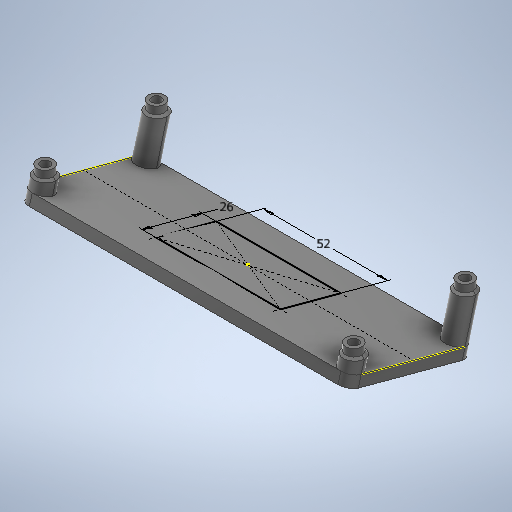
# Autodesk Inventor part: relay_module_standoffs_angled_plate
Saved by Autodesk Inventor 2025.1 (Build 291241000, 241)
## iProperties
Created: 2026-06-20
Part Number: relay_module_standoffs_angled_plate
Material: Generic
Document SubType Name: Modeling
Designer: Aiden
Density: 1 g/cm^3
Appearance: Default
Author: Aiden
Autodesk Inventor part; units mm, degrees
ref_plane "YZ Plane" through (0, 0, 0) normal (1, 0, 0) x (0, 1, 0)
ref_plane "XZ Plane" through (0, 0, 0) normal (0, 1, 0) x (-1, 0, 0)
ref_plane "XY Plane" through (0, 0, 0) normal (0, 0, 1) x (1, 0, 0)
sketch "Relay Hole Layout" plane through (0, 0, 0) normal (0, 1, 0) x (-1, 0, 0)
  line L0 (64.4668, 23.2607) -> (-64.4668, 23.2607) construction
  line L1 (-64.4668, 23.2607) -> (-64.4668, -23.2607) construction
  line L2 (-64.4668, -23.2607) -> (64.4668, -23.2607) construction
  line L3 (64.4668, -23.2607) -> (64.4668, 23.2607) construction
  line L4 (64.4668, 23.2607) -> (-64.4668, -23.2607) construction
  line L5 (-64.4668, 23.2607) -> (64.4668, -23.2607) construction
  circle A0 centre (64.4668, -23.2607) radius 1.625 construction
  line L6 (0, -23.2607) -> (0, 23.2607) construction
  line L7 (64.4668, 0) -> (-64.4668, 0) construction
  circle A1 centre (-64.4668, -23.2607) radius 1.625 construction
  circle A2 centre (64.4668, 23.2607) radius 1.625 construction
  circle A3 centre (-64.4668, 23.2607) radius 1.625 construction
  line L8 (67.4918, -26.2857) -> (-67.4918, -26.2857) construction
  line L9 (-67.4918, -26.2857) -> (-67.4918, 26.2857) construction
  line L10 (-67.4918, 26.2857) -> (67.4918, 26.2857) construction
  line L11 (67.4918, 26.2857) -> (67.4918, -26.2857) construction
  line L12 (66.0918, -23.2607) -> (67.4918, -23.2607) construction
  line L13 (-64.4668, 24.8857) -> (-64.4668, 26.2857) construction
  line L14 (-66.0918, 23.2607) -> (-67.4918, 23.2607) construction
  point P0 (0, 0)
  dimension "d2" = 3.25
  dimension "d0" = 46.5214
  dimension "d1" = 128.9336
  dimension "d5" = 1.4
  dimension "d6" = 1.4
  dimension "d7" = 1.4
  dimension "d8" = 1.4
  constraints: 30 end point, 6 midpoint, 5 perpendicular, 4 parallel, 3 centre point, 3 point on line, 3 symmetric about line, 2 horizontal, 2 point on circle, 1 coincident, 1 horizontal alignment, 5 other
  measures "d0" distance of L2.end L0.start
  measures "d1" distance of L1.end L2.end
  measures "d6" distance of L12.start L12.end
  measures "d7" distance of L14.start L14.end
  measures "d8" distance of L13.start L13.end
sketch "Sketch2" plane through (0, 0, 0) normal (0, 1, 0) x (-1, 0, 0)
  circle A0 centre (64.4668, -23.2607) radius 1.625 construction
  circle A1 centre (-64.4668, -23.2607) radius 1.625 construction
  circle A2 centre (-64.4668, 23.2607) radius 1.625 construction
  circle A3 centre (64.4668, 23.2607) radius 1.625 construction
  circle A4 centre (64.4668, -23.2607) radius 3.375
  circle A5 centre (-64.4668, -23.2607) radius 3.375
  circle A6 centre (-64.4668, 23.2607) radius 3.375
  circle A7 centre (64.4668, 23.2607) radius 3.375
  point P0 (0, 0)
  dimension "d9" = 1.75
  constraints: 4 centre point, 4 coincident, 3 equal radius
  measures "d9" radial gap between concentric circles of A4 A0
extrude "Extrusion2" add sketch "Sketch2" along normal blind 4
sketch "Sketch3" plane through (-64.4668, 4, -23.2607) normal (0, 1, 0) x (1, 0, 0)
  circle A0 centre (0, 0) radius 3.375 projected
  circle A1 centre (128.9336, 0) radius 3.375 projected
  circle A2 centre (128.9336, -46.5214) radius 3.375 projected
  circle A3 centre (0, -46.5214) radius 3.375 projected
  point P0 (64.4668, -23.2607)
  constraints: 4 coincident
hole "Hole1" at (-64.4668, 4, -23.2607) at (64.4668, 4, -23.2607) at (64.4668, 4, 23.2607) at (-64.4668, 4, 23.2607) direction (0, -1, 0) diameter 4 depth 3
ref_plane "Work Plane1" through (0, 0, 0) normal (0, 1, 0) x (1, 0, 0)
sketch "Sketch4" plane through (-64.4668, 0, -23.2607) normal (0, -1, 0) x (1, 0, 0)
  circle A0 centre (0, 0) radius 2 construction
  circle A1 centre (0, 46.5214) radius 2 construction
  circle A2 centre (128.9336, 46.5214) radius 3.375 construction
  circle A3 centre (128.9336, 0) radius 2 construction
  line L0 (0, 0) -> (128.9336, 0) construction
  circle A4 centre (0, 46.5214) radius 3.375 construction
  line L1 (0, 46.5214) -> (128.9336, 46.5214) construction
  point P0 (64.4668, 23.2607)
  constraints: 4 coincident, 4 end point, 2 horizontal
ref_plane "Work Plane3" through (-64.4668, -16.4811, -18.8446) normal (0, -0.9659258, 0.258819) x (1, 0, 0)
ref_plane "Work Plane2" through (-64.4668, 0, -23.2607) normal (0, -0.9659258, 0.258819) x (1, 0, 0)
sketch "Sketch5" plane through (-64.4668, -16.4811, -18.8446) normal (0, -0.9659258, 0.258819) x (1, 0, 0)
  ellipse E0 centre (0, 44.9362) end of major axis (-3.375, 44.9362) minor radius 3.26 projected
  ellipse E1 centre (0, 0) end of major axis (-3.375, 0) minor radius 3.26 projected
  ellipse E2 centre (128.9336, 44.9362) end of major axis (125.5586, 44.9362) minor radius 3.26 projected
  ellipse E3 centre (128.9336, 0) end of major axis (125.5586, 0) minor radius 3.26 projected
  point P0 (64.4668, 22.4681)
  constraints: 4 other
extrude "Extrusion3" add sketch "Sketch5" against normal up to surface contours E0 | E2 surface through (64.4668, 0, -23.2607) normal (0, 1, 0)
sketch "Sketch6" plane through (-64.4668, -16.4811, -18.8446) normal (0, -0.9659258, 0.258819) x (1, 0, 0)
  ellipse E0 centre (128.9336, 0) end of major axis (125.5586, 0) minor radius 3.26 projected
  ellipse E1 centre (0, 0) end of major axis (-3.375, 0) minor radius 3.26 projected
  point P0 (64.4668, 22.4681)
  constraints: 2 other
extrude "Extrusion4" add sketch "Sketch6" against normal up to surface surface through (64.4668, 0, -23.2607) normal (0, 1, 0)
thicken "Thicken1" operation add thickness 1 both sides no extend neighbours no toward (-0.0100441, -0.258806, -0.9658771) faces at (-64.5019, -5.779, -25.087)
thicken "Thicken2" operation add thickness 1 both sides no extend neighbours no toward (-0.0100441, -0.258806, -0.9658771) faces at (-64.5019, -1.9022, 20.3956)
thicken "Thicken3" operation add thickness 1 both sides no extend neighbours no toward (-0.0100441, -0.258806, -0.9658771) faces at (64.4317, -5.779, -25.087)
thicken "Thicken4" operation add thickness 1 both sides no extend neighbours no toward (-0.010044, -0.258806, -0.9658771) faces at (64.4317, -1.9022, 20.3956)
chamfer "Chamfer2" distance 1 angle 45 4 edges at (-61.0918, 0, 23.2607) (-61.0918, 0, -23.2607) (67.8418, 0, -23.2607) (67.8418, 0, 23.2607)
sketch "Sketch7" plane through (-64.4668, 1, -23.2607) normal (0, 1, 0) x (1, 0, 0)
  circle A0 centre (0, 0) radius 2 projected
  circle A1 centre (0, -46.5214) radius 2 projected
  circle A2 centre (128.9336, -46.5214) radius 2 projected
  circle A3 centre (128.9336, 0) radius 2 projected
  point P0 (64.4668, -23.2607)
extrude "Extrusion5" cut sketch "Sketch7" against normal blind 5 from surface at 3
sketch "Sketch8" plane through (-64.4668, -16.4811, -18.8446) normal (0, -0.9659258, 0.258819) x (1, 0, 0)
  line L0 (133.3086, 49.1962) -> (-4.375, 49.1962)
  line L1 (-4.375, 49.1962) -> (-4.375, -4.26)
  line L2 (-4.375, -4.26) -> (133.3086, -4.26)
  line L3 (133.3086, -4.26) -> (133.3086, 49.1962)
  spline S0 degree 12 poles (124.5586, 44.9362) (124.5586, 43.8117) (124.8911, 42.6872) (125.5559, 41.669) (126.5121, 40.8623) (127.6713, 40.3548) (128.9336, 40.1771) (130.1959, 40.3548) (131.3551, 40.8623) (132.3113, 41.669) (132.9761, 42.6872) (133.3086, 43.8117) (133.3086, 46.0607) (132.9761, 47.1852) (132.3113, 48.2035) (131.3551, 49.0102) (130.1959, 49.5176) (128.9336, 49.6953) (127.6713, 49.5176) (126.5121, 49.0102) (125.5559, 48.2035) (124.8911, 47.1852) (124.5586, 46.0607) (124.5586, 44.9362) knots 0 0 0 0 0 0 0 0 0 0 0 0 0 0.5 0.5 0.5 0.5 0.5 0.5 0.5 0.5 0.5 0.5 0.5 1 1 1 1 1 1 1 1 1 1 1 1 1 projected
  spline S1 degree 12 poles (124.5586, 0) (124.5586, -1.1245) (124.8911, -2.249) (125.5559, -3.2673) (126.5121, -4.0739) (127.6713, -4.5814) (128.9336, -4.7591) (130.1959, -4.5814) (131.3551, -4.0739) (132.3113, -3.2673) (132.9761, -2.249) (133.3086, -1.1245) (133.3086, 1.1245) (132.9761, 2.249) (132.3113, 3.2673) (131.3551, 4.0739) (130.1959, 4.5814) (128.9336, 4.7591) (127.6713, 4.5814) (126.5121, 4.0739) (125.5559, 3.2673) (124.8911, 2.249) (124.5586, 1.1245) (124.5586, 0) knots 0 0 0 0 0 0 0 0 0 0 0 0 0 0.5 0.5 0.5 0.5 0.5 0.5 0.5 0.5 0.5 0.5 0.5 1 1 1 1 1 1 1 1 1 1 1 1 1 projected
  spline S2 degree 12 poles (-4.375, 0) (-4.375, -1.1245) (-4.0425, -2.249) (-3.3777, -3.2673) (-2.4215, -4.0739) (-1.2623, -4.5814) (0, -4.7591) (1.2623, -4.5814) (2.4215, -4.0739) (3.3777, -3.2673) (4.0425, -2.249) (4.375, -1.1245) (4.375, 1.1245) (4.0425, 2.249) (3.3777, 3.2673) (2.4215, 4.0739) (1.2623, 4.5814) (0, 4.7591) (-1.2623, 4.5814) (-2.4215, 4.0739) (-3.3777, 3.2673) (-4.0425, 2.249) (-4.375, 1.1245) (-4.375, 0) knots 0 0 0 0 0 0 0 0 0 0 0 0 0 0.5 0.5 0.5 0.5 0.5 0.5 0.5 0.5 0.5 0.5 0.5 1 1 1 1 1 1 1 1 1 1 1 1 1 projected
  spline S3 degree 12 poles (-4.375, 44.9362) (-4.375, 43.8117) (-4.0425, 42.6872) (-3.3777, 41.669) (-2.4215, 40.8623) (-1.2623, 40.3548) (0, 40.1771) (1.2623, 40.3548) (2.4215, 40.8623) (3.3777, 41.669) (4.0425, 42.6872) (4.375, 43.8117) (4.375, 46.0607) (4.0425, 47.1852) (3.3777, 48.2035) (2.4215, 49.0102) (1.2623, 49.5176) (0, 49.6953) (-1.2623, 49.5176) (-2.4215, 49.0102) (-3.3777, 48.2035) (-4.0425, 47.1852) (-4.375, 46.0607) (-4.375, 44.9362) knots 0 0 0 0 0 0 0 0 0 0 0 0 0 0.5 0.5 0.5 0.5 0.5 0.5 0.5 0.5 0.5 0.5 0.5 1 1 1 1 1 1 1 1 1 1 1 1 1 projected
  point P0 (64.4668, 22.4681)
  point P1 (-4.375, 44.9362)
  point P2 (-4.375, 0)
  point P3 (0, -4.26)
  point P4 (128.9336, -4.26)
  point P5 (128.9336, 49.1962)
  point P6 (0, 49.1962)
  constraints: 8 end point, 3 horizontal, 2 parallel, 2 vertical, 1 perpendicular, 4 other
extrude "Extrusion6" add sketch "Sketch8" along normal blind 4.5 contours S0 L3 S1 L2 S2 L1 S3 L0 | S0 | S3 | S1 | S2
sketch "Sketch9" plane through (-64.4668, -16.4811, -18.8446) normal (0, 0.9659258, -0.258819) x (1, 0, 0)
  point P0 (64.4668, -22.4681)
sketch "Sketch10" plane through (-64.4668, -16.4811, -18.8446) normal (0, 0.9659258, -0.258819) x (1, 0, 0)
  line L0 (-4.375, -44.9362) -> (-4.375, 0) projected
  line L1 (-4.375, -22.4681) -> (133.3086, -22.4681) construction
  line L2 (133.3086, 0) -> (133.3086, -44.9362) projected
  line L3 (90.4668, -35.4681) -> (38.4668, -35.4681)
  line L4 (38.4668, -35.4681) -> (38.4668, -9.4681)
  line L5 (38.4668, -9.4681) -> (90.4668, -9.4681)
  line L6 (90.4668, -9.4681) -> (90.4668, -35.4681)
  line L7 (90.4668, -35.4681) -> (38.4668, -9.4681) construction
  line L8 (38.4668, -35.4681) -> (90.4668, -9.4681) construction
  point P0 (64.4668, -22.4681)
  dimension "d43" = 52
  dimension "d44" = 26
  constraints: 14 end point, 4 coincident, 4 midpoint, 2 parallel, 1 horizontal, 1 perpendicular
  measures "d43" distance of L4.end L5.end
  measures "d44" distance of L3.end L4.end
body "Solid2"
